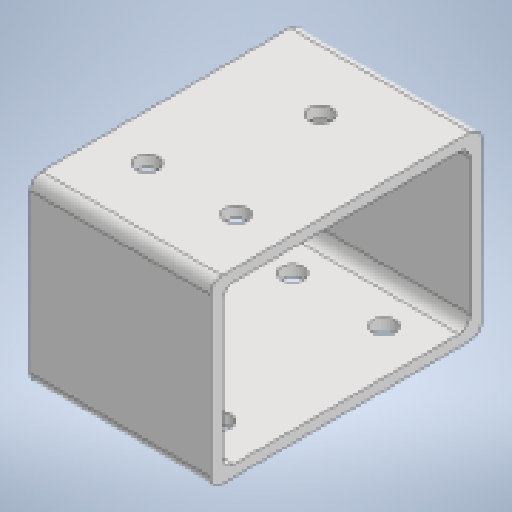
# Autodesk Inventor part: 3x2_Bar
Saved by Autodesk Inventor 2023 (Build 270158000, 158)
## iProperties
Created: 2025-04-19
Part Number: 3x2_Bar
Material: Generic
Document SubType Name: Modeling
Designer: plebbb
Density: 1 g/cm^3
Appearance: Default
Author: plebbb
Autodesk Inventor part; units mm, degrees
ref_plane "YZ Plane" through (0, 0, 0) normal (1, 0, 0) x (0, 1, 0)
ref_plane "XZ Plane" through (0, 0, 0) normal (0, 1, 0) x (-1, 0, 0)
ref_plane "XY Plane" through (0, 0, 0) normal (0, 0, 1) x (1, 0, 0)
sketch "Sketch1" plane through (0, 0, 0) normal (1, 0, 0) x (0, 1, 0)
  line L0 (0, 0) -> (50.8, 0)
  line L1 (50.8, 0) -> (50.8, -76.2)
  line L2 (50.8, -76.2) -> (0, -76.2)
  line L3 (0, -76.2) -> (0, 0)
  dimension "d0" = 76.2
  dimension "d1" = 50.8
  constraints: 8 end point, 2 parallel, 1 horizontal, 1 perpendicular
  measures "d0" distance of L0.end L1.end
  measures "d1" distance of L1.end L2.end
extrude "Extrusion1" add sketch "Sketch1" along normal blind 50.8
shell "Shell1" thickness 3.175 removed faces 2 at (50.8, 33.8667, -50.8) at (0, 33.8667, -50.8)
fillet "Fillet1" radius 3.175 8 edges at (25.4, 47.625, -3.175) (25.4, 50.8, 0) (25.4, 3.175, -3.175) (25.4, 0, 0) (25.4, 50.8, -76.2) (25.4, 47.625, -73.025) (25.4, 3.175, -73.025) (25.4, 0, -76.2)
sketch "Sketch2" plane through (0, 0, -73.025) normal (0, -1, 0) x (1, 0, 0)
  circle A0 centre (12.5, 11.825) radius 3.175
  circle A1 centre (12.5, 58.025) radius 3.175
  circle A2 centre (38.3, 11.825) radius 3.175
  circle A3 centre (38.3, 58.025) radius 3.175
  line L0 (12.5, 11.825) -> (38.3, 11.825) construction
  line L1 (38.3, 11.825) -> (38.3, 58.025) construction
  line L2 (38.3, 58.025) -> (12.5, 58.025) construction
  line L3 (12.5, 58.025) -> (12.5, 11.825) construction
  line L4 (0, 73.025) -> (50.8, 73.025) construction
  line L5 (50.8, 73.025) -> (50.8, -3.175) construction
  line L6 (50.8, -3.175) -> (0, -3.175) construction
  line L7 (0, -3.175) -> (0, 73.025) construction
  point P0 (25.4, 58.025)
  point P1 (25.4, 73.025)
  point P2 (12.5, 34.925)
  point P3 (0, 34.925)
  dimension "d6" = 6.35
  dimension "d7" = 50.8
  dimension "d8" = 76.2
  dimension "d10" = 12.5
  dimension "d11" = 15
  constraints: 16 end point, 4 centre point, 4 midpoint, 4 parallel, 3 equal radius, 2 coincident, 2 horizontal, 2 perpendicular, 1 horizontal alignment, 1 vertical alignment
  measures "d6" diameter of A0
  measures "d7" distance of L4.start L4.end
  measures "d8" distance of L6.end L4.start
  measures "d10" distance of point (0, 34.925) point (12.5, 34.925)
  measures "d11" distance between parallel lines of L4 L2
extrude "Extrusion2" cut sketch "Sketch2" against normal up to surface (3.175 mm away)
sketch "Sketch3" plane through (0, 50.8, -3.175) normal (0, 1, 0) x (1, 0, 0)
  line L0 (0, -3.175) -> (50.8, -3.175) construction
  line L1 (50.8, -3.175) -> (50.8, 73.025) construction
  line L2 (50.8, 73.025) -> (0, 73.025) construction
  line L3 (0, 73.025) -> (0, -3.175) construction
  line L4 (47.625, 73.025) -> (47.625, -3.175) construction
  line L5 (3.175, -3.175) -> (3.175, 73.025) construction
  line L6 (47.625, 34.925) -> (50.8, 34.925) construction
  line L7 (3.175, 34.925) -> (0, 34.925) construction
  line L8 (37.9, 53.025) -> (12.9, 53.025) construction
  line L9 (12.9, 53.025) -> (12.9, 16.825) construction
  line L10 (12.9, 16.825) -> (37.9, 16.825) construction
  line L11 (37.9, 16.825) -> (37.9, 53.025) construction
  circle A0 centre (25.4, 53.025) radius 3.175
  circle A1 centre (12.9, 16.825) radius 3.175
  circle A2 centre (37.9, 16.825) radius 3.175
  line L12 (25.4, 16.825) -> (25.4, -3.175) construction
  line L13 (25.4, 53.025) -> (25.4, 73.025) construction
  dimension "d14" = 3.175
  dimension "d15" = 76.2
  dimension "d16" = 50.8
  dimension "d17" = 6.35
  dimension "d19" = 25
  dimension "d20" = 20
  constraints: 28 end point, 8 midpoint, 4 parallel, 4 perpendicular, 4 point on line, 3 centre point, 2 coincident, 2 collinear, 2 equal radius, 2 horizontal
  measures "d14" distance of L6.start L6.end
  measures "d15" distance of L0.end L1.end
  measures "d16" distance of L0.start L0.end
  measures "d17" diameter of A2
  measures "d19" distance of L9.end L10.end
  measures "d20" distance of L13.start L13.end
extrude "Extrusion3" cut sketch "Sketch3" against normal up to surface (3.175 mm away)
body "Solid1"
